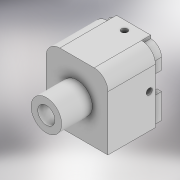
# Autodesk Inventor part: Cap_Holder
Saved by Autodesk Inventor 2020 (Build 240168000, 168)
## iProperties
Created: 2022-04-06
Part Number: Cap_Holder
Material: 일반
Document SubType Name: Modeling
Designer: Knowblesse
Density: 1 g/cm^3
Appearance: 기본값
Author: Knowblesse
## iProperties of the stored document _3D 인쇄.ipt
Created: 2022-04-06
Part Number: _3D 인쇄
Material: 일반
Document SubType Name: Modeling
Designer: Knowblesse
Density: 1 g/cm^3
Appearance: 기본값
Author: Knowblesse
Autodesk Inventor part; units mm, degrees
ref_plane "YZ Plane" through (0, 0, 0) normal (1, 0, 0) x (0, 1, 0)
ref_plane "XZ Plane" through (0, 0, 0) normal (0, 1, 0) x (-1, 0, 0)
ref_plane "XY Plane" through (0, 0, 0) normal (0, 0, 1) x (1, 0, 0)
sketch "스케치1" plane through (0, 0, 0) normal (0, 0, 1) x (1, 0, 0)
  line L0 (-5.6, -8.7) -> (7.6, -8.7)
  line L1 (7.6, -8.7) -> (7.6, 6.7)
  line L2 (5.6, 8.7) -> (-5.6, 8.7)
  line L3 (-7.6, 6.7) -> (-7.6, -6.7)
  line L4 (-7.6, -8.7) -> (7.6, 8.7) construction
  line L5 (7.6, -8.7) -> (-7.6, 8.7) construction
  arc A0 (-5.6, 8.7) -> (-7.6, 6.7) centre (-5.6, 6.7) ccw
  arc A1 (7.6, 6.7) -> (5.6, 8.7) centre (5.6, 6.7) ccw
  arc A2 (-7.6, -6.7) -> (-5.6, -8.7) centre (-5.6, -6.7) ccw
  line L6 (-5.6, 10.2) -> (5.6, 10.2)
  arc A3 (9.1, 6.7) -> (5.6, 10.2) centre (5.6, 6.7) ccw
  line L7 (9.1, 6.7) -> (9.1, -10.2)
  line L8 (9.1, -10.2) -> (-5.6, -10.2)
  arc A4 (-9.1, -6.7) -> (-5.6, -10.2) centre (-5.6, -6.7) ccw
  line L9 (-9.1, -6.7) -> (-9.1, 6.7)
  arc A5 (-5.6, 10.2) -> (-9.1, 6.7) centre (-5.6, 6.7) ccw
  point P0 (0, 0)
  dimension "d0" = 17.4
  dimension "d1" = 15.2
  dimension "d2" = 2
  dimension "d3" = 1.5
  constraints: 20 end point, 12 point on circle, 6 centre point, 6 point on line, 6 tangent, 4 parallel, 2 equal radius, 2 midpoint, 2 perpendicular, 1 horizontal, 6 other
  measures "d0" distance of L0.end L4.end
  measures "d1" distance of L4.end L5.end
  measures "d2" radius of A0
  measures "d3" distance between parallel lines of L2 L6
extrude "돌출1" add sketch "스케치1" along normal blind 17
sketch "스케치2" plane through (0, 0, 17) normal (0, 0, 1) x (1, 0, 0)
  line L0 (-5.6, -10.2) -> (9.1, -10.2) projected
  line L1 (9.1, -10.2) -> (9.1, 6.7) projected
  arc A0 (9.1, 6.7) -> (5.6, 10.2) centre (5.6, 6.7) ccw projected
  line L2 (5.6, 10.2) -> (-5.6, 10.2) projected
  arc A1 (-5.6, 10.2) -> (-9.1, 6.7) centre (-5.6, 6.7) ccw projected
  line L3 (-9.1, 6.7) -> (-9.1, -6.7) projected
  arc A2 (-9.1, -6.7) -> (-5.6, -10.2) centre (-5.6, -6.7) ccw projected
  point P0 (0, 0)
extrude "돌출2" add sketch "스케치2" along normal blind 1.5
sketch "스케치3" plane through (-9.1, -6.7, 0) normal (-1, 0, 0) x (0, 0, 1)
  line L0 (0, 13.4) -> (0, 0) projected
  line L1 (3, 3.7) -> (1.5, 3.7)
  line L2 (1.5, 3.7) -> (1.5, 9.7)
  line L3 (1.5, 9.7) -> (3, 9.7)
  line L4 (3, 9.7) -> (3, 3.7)
  point P0 (0, 6.7)
  point P1 (0, 6.7)
  point P2 (1.5, 6.7)
  dimension "d8" = 6
  dimension "d9" = 1.5
  dimension "d10" = 1.5
  constraints: 8 end point, 2 midpoint, 2 parallel, 1 horizontal, 1 horizontal alignment, 1 perpendicular
  measures "d8" distance of L1.end L2.end
  measures "d9" distance of L2.end L3.end
  measures "d10" distance between parallel lines of L2 L0
extrude "돌출3" cut sketch "스케치3" against normal through all
sketch "스케치6" plane through (0, 0, 18.5) normal (0, 0, 1) x (1, 0, 0)
  arc A0 (-9.1, -6.7) -> (-5.6, -10.2) centre (-5.6, -6.7) ccw projected
  line L0 (-5.6, -10.2) -> (9.1, -10.2) projected
  line L1 (9.1, -10.2) -> (9.1, 6.7) projected
  arc A1 (9.1, 6.7) -> (5.6, 10.2) centre (5.6, 6.7) ccw projected
  line L2 (5.6, 10.2) -> (-5.6, 10.2) projected
  arc A2 (-5.6, 10.2) -> (-9.1, 6.7) centre (-5.6, 6.7) ccw projected
  line L3 (-9.1, 6.7) -> (-9.1, -6.7) projected
  arc A3 (-10.1, -6.7) -> (-5.6, -11.2) centre (-5.6, -6.7) ccw
  line L4 (-5.6, -11.2) -> (10.1, -11.2)
  line L5 (10.1, -11.2) -> (10.1, 6.7)
  arc A4 (10.1, 6.7) -> (5.6, 11.2) centre (5.6, 6.7) ccw
  line L6 (5.6, 11.2) -> (-5.6, 11.2)
  arc A5 (-5.6, 11.2) -> (-10.1, 6.7) centre (-5.6, 6.7) ccw
  line L7 (-10.1, 6.7) -> (-10.1, -6.7)
  point P0 (0, 0)
  dimension "d23" = 1
  constraints: 8 end point, 6 point on circle, 3 centre point, 6 other
  measures "d23" distance between parallel lines of L3 L7
extrude "돌출5" add sketch "스케치6" against normal blind 15.5
sketch "스케치7" plane through (-5.6, -10.2, 0) normal (0, -1, 0) x (1, 0, 0)
  line L0 (14.7, 3) -> (0, 3) projected
  line L1 (0, 0) -> (0, 3) projected
  line L2 (0, 0) -> (14.7, 0) projected
  line L3 (14.7, 0) -> (14.7, 3) projected
  point P0 (5.6, 0)
extrude "돌출6" add sketch "스케치7" along normal up to surface (1 mm away)
sketch "스케치8" plane through (-5.6, 10.2, 0) normal (0, 1, 0) x (1, 0, 0)
  line L0 (0, -3) -> (11.2, -3) projected
  line L1 (11.2, 0) -> (11.2, -3) projected
  line L2 (11.2, 0) -> (0, 0) projected
  line L3 (0, 0) -> (0, -3) projected
  point P0 (5.6, 0)
extrude "돌출7" add sketch "스케치8" along normal up to surface (1 mm away)
sketch "스케치9" plane through (-5.6, -11.2, 18.5) normal (0, -1, 0) x (1, 0, 0)
  line L0 (15.7, -15.5) -> (14.7, -15.5) projected
  point P0 (5.6, -18.5)
  point P1 (5.6, -15.5)
  point P2 (15.2, -15.5)
  constraints: 1 horizontal alignment, 1 midpoint, 1 vertical alignment
hole "구멍1" at (0, -11.2, 3) direction (0, 1, 0) diameter 2 end through all
sketch "스케치10" plane through (7.6, -3, 1.5) normal (0, 0, 1) x (1, 0, 0)
  line L0 (0, 0) -> (0, 6) projected
  line L1 (0, 0) -> (1.5, 0) projected
  line L2 (1.5, 6) -> (1.5, 0) projected
  line L3 (0, 6) -> (1.5, 6) projected
  arc A0 (0, 9.7) -> (-2, 11.7) centre (-2, 9.7) ccw projected
  line L4 (-2, 11.7) -> (-13.2, 11.7) projected
  arc A1 (-13.2, 11.7) -> (-15.2, 9.7) centre (-13.2, 9.7) ccw projected
  line L5 (-15.2, 9.7) -> (-15.2, 6) projected
  line L6 (-15.2, 6) -> (-16.7, 6) projected
  line L7 (-16.7, 6) -> (-16.7, 9.7) projected
  arc A2 (-13.2, 13.2) -> (-16.7, 9.7) centre (-13.2, 9.7) ccw projected
  line L8 (-13.2, 13.2) -> (-13.2, 14.2) projected
  line L9 (-13.2, 14.2) -> (-2, 14.2) projected
  line L10 (-2, 14.2) -> (-2, 13.2) projected
  arc A3 (1.5, 9.7) -> (-2, 13.2) centre (-2, 9.7) ccw projected
  line L11 (1.5, 9.7) -> (1.5, 6) projected
  line L12 (1.5, 6) -> (1.5, 0) projected
  line L13 (0, 0) -> (1.5, 0) projected
  line L14 (0, -5.7) -> (0, 0) projected
  line L15 (-13.2, -5.7) -> (0, -5.7) projected
  arc A4 (-15.2, -3.7) -> (-13.2, -5.7) centre (-13.2, -3.7) ccw projected
  line L16 (-15.2, 0) -> (-15.2, -3.7) projected
  line L17 (-15.2, 6) -> (-15.2, 0) projected
  line L18 (0, 6) -> (0, 9.7) projected
  line L19 (1.5, 6) -> (0, 6) projected
  line L20 (-16.7, 0) -> (-16.7, 6) projected
  line L21 (-16.7, -3.7) -> (-16.7, 0) projected
  arc A5 (-16.7, -3.7) -> (-13.2, -7.2) centre (-13.2, -3.7) ccw projected
  line L22 (-13.2, -8.2) -> (-13.2, -7.2) projected
  line L23 (1.5, -8.2) -> (-13.2, -8.2) projected
  line L24 (1.5, 0) -> (1.5, -8.2) projected
  line L25 (0, 0) -> (0, 6) projected
  line L26 (-16.7, 0) -> (-15.2, 0) projected
  point P0 (-7.6, 3)
extrude "돌출8" cut sketch "스케치10" against normal blind 15.5 contours L0 L3 L2 L1 | L26 L20 L6 L17
sketch "스케치11" plane through (10.1, -11.2, 18.5) normal (1, 0, 0) x (0, 0, -1)
  line L0 (15.5, 17.9) -> (15.5, 0) projected
  point P0 (18.5, 11.2)
  point P1 (13.5, 11.2)
  dimension "d39" = 2
  constraints: 1 horizontal alignment
  measures "d39" distance from line of point (13.5, 11.2) L0
hole "구멍2" at (10.1, 0, 5) direction (-1, 0, 0) diameter 2 end through all
sketch "스케치13" plane through (0, 0, 18.5) normal (0, 0, 1) x (1, 0, 0)
  circle A0 centre (0, 0) radius 5
  dimension "d47" = 10
  constraints: 1 centre point, 1 coincident
  measures "d47" diameter of A0
extrude "돌출9" add sketch "스케치13" along normal blind 10
sketch "스케치14" plane through (0, 0, 28.5) normal (0, 0, 1) x (1, 0, 0)
  circle A0 centre (0, 0) radius 5 projected
  circle A1 centre (0, 0) radius 2.8
  dimension "d50" = 5.6
  constraints: 1 centre point, 1 coincident
  measures "d50" diameter of A1
extrude "돌출10" cut sketch "스케치14" against normal blind 7 contours A1
sketch "스케치15" plane through (0, 0, 21.5) normal (0, 0, 1) x (1, 0, 0)
  circle A0 centre (0, 0) radius 2.8 projected
  circle A1 centre (0, 0) radius 1.5
  dimension "d53" = 3
  constraints: 1 centre point, 1 coincident
  measures "d53" diameter of A1
extrude "돌출11" cut sketch "스케치15" against normal through all contours A1
sketch "스케치16" plane through (0, 0, 17) normal (0, 0, -1) x (-1, 0, 0)
  circle A0 centre (0, 0) radius 1.5 projected
  circle A1 centre (0, 0) radius 3
  dimension "d56" = 6
  constraints: 1 centre point, 1 coincident
  measures "d56" diameter of A1
extrude "돌출12" cut sketch "스케치16" against normal blind 3
